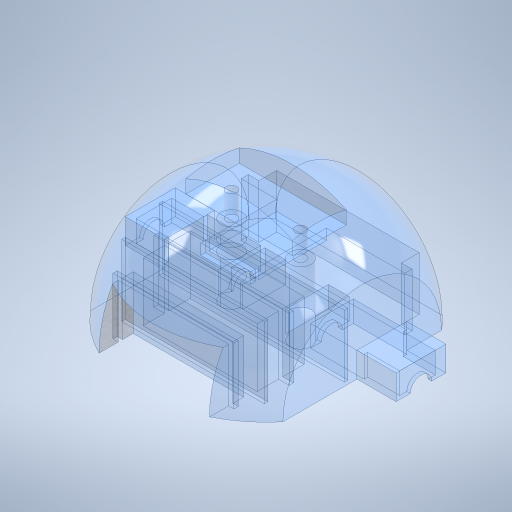
# Autodesk Inventor part: naibu-rightside
Saved by Autodesk Inventor 2023 (Build 270158000, 158)
## iProperties
Created: 2022-10-08
Part Number: naibu-rightside
Material: ABS プラスチック
Document SubType Name: Modeling
Designer: ellie
Density: 1.06 g/cm^3
Appearance: 青 - 光沢
Author: ellie
Autodesk Inventor part; units mm, degrees
ref_plane "YZ Plane" through (0, 0, 0) normal (1, 0, 0) x (0, 1, 0)
sketch "スケッチ1" plane through (0, 0, 0) normal (0, 1, 0) x (-1, 0, 0)
  circle A0 centre (0, 0) radius 35
  line L0 (0, 0) -> (0, -35)
  line L1 (0, 0) -> (0, 35)
  dimension "d0" = 70
  constraints: 4 end point, 2 point on circle, 2 vertical, 1 centre point, 1 coincident
  measures "d0" diameter of A0
revolve "回転1" add sketch "スケッチ1" angle 180 about axis through (0, 0, 0) along (0, 0, 1) picked at (-2.5961, -23.0408) contours L1 L0 A0
sketch "スケッチ5" plane through (0, 0, 0) normal (0, -1, 0) x (1, 0, 0)
  line L0 (-20, -23) -> (20, -23)
  line L1 (20, -23) -> (20, -16)
  line L2 (20, -16) -> (-20, -16)
  line L3 (-20, -16) -> (-20, -23)
  line L4 (-20, -16) -> (-23, -16)
  line L5 (-23, -16) -> (-23, -18)
  line L6 (-23, -18) -> (-20, -18)
  line L7 (-20, -18) -> (-20, -16)
  line L8 (0, 26) -> (-17, 26)
  line L9 (-17, 26) -> (-17, 24.8)
  line L10 (-17, 24.8) -> (0, 24.8)
  line L11 (0, 24.8) -> (0, 26)
  line L12 (0, 20.5) -> (-20, 20.5)
  line L13 (-20, 20.5) -> (-20, 19.5)
  line L14 (-20, 19.5) -> (0, 19.5)
  line L15 (0, 19.5) -> (0, 20.5)
  line L16 (0, 12.5) -> (-19, 12.5)
  line L17 (-19, 12.5) -> (-19, 11.3)
  line L18 (-19, 11.3) -> (0, 11.3)
  line L19 (0, 11.3) -> (0, 12.5)
  line L20 (0, 4) -> (-26, 4)
  line L21 (-26, 4) -> (-26, 3)
  line L22 (-26, 3) -> (0, 3)
  line L23 (0, 3) -> (0, 4)
  circle A0 centre (0, 0) radius 35 projected
  circle A1 centre (0, 0) radius 35 projected
  line L24 (0, 35) -> (0, -35)
  line L25 (35, 0) -> (-35, 0)
  line L26 (-37, -0.5262) -> (-28, -0.5262)
  line L27 (-28, -0.5262) -> (-28, -10.5262)
  line L28 (-28, -10.5262) -> (-37, -10.5262)
  line L29 (-37, -10.5262) -> (-37, -0.5262)
  line L30 (-28, -8.0262) -> (-28, -0.5262)
  line L31 (-27, 22.2711) -> (-27, -22.2711)
  line L32 (-15.5, 26) -> (0, 26)
  line L33 (0, 26) -> (0, 35)
  line L34 (0, 35) -> (-15.5, 35)
  line L35 (-15.5, 35) -> (-15.5, 26)
  line L36 (-15.5, 24.8) -> (0, 24.8)
  line L37 (0, 24.8) -> (0, 21.8)
  line L38 (0, 21.8) -> (-15.5, 21.8)
  line L39 (-15.5, 21.8) -> (-15.5, 24.8)
  line L40 (-16, 12.5) -> (0, 12.5)
  line L41 (0, 12.5) -> (0, 18.5)
  line L42 (0, 18.5) -> (-16, 18.5)
  line L43 (-16, 18.5) -> (-16, 12.5)
  line L44 (-16, 11.3) -> (0, 11.3)
  line L45 (0, 11.3) -> (0, 5.3)
  line L46 (0, 5.3) -> (-16, 5.3)
  line L47 (-16, 5.3) -> (-16, 11.3)
  line L48 (-28, -5.5262) -> (-44.6865, -5.5262)
  line L49 (-28, -5.5262) -> (-12.8337, -5.5262)
  line L50 (-13, 0.4738) -> (-28, 0.4738)
  line L51 (-28, 0.4738) -> (-28, -11.5262)
  line L52 (-28, -11.5262) -> (-13, -11.5262)
  line L53 (-13, -11.5262) -> (-13, 0.4738)
  line L54 (-13, 0.4738) -> (-28, -11.5262) construction
  line L55 (-28, 0.4738) -> (-13, -11.5262) construction
  line L56 (-28, 1.4738) -> (-38, 1.4738)
  line L57 (-38, 1.4738) -> (-38, -12.5262)
  line L58 (-38, -12.5262) -> (-28, -12.5262)
  line L59 (-28, -12.5262) -> (-28, 1.4738)
  line L60 (-28, 1.4738) -> (-38, -12.5262) construction
  line L61 (-38, 1.4738) -> (-28, -12.5262) construction
  line L62 (-13, 0.4738) -> (-6, 0.4738)
  line L63 (-6, 0.4738) -> (-6, -11.5262)
  line L64 (-6, -11.5262) -> (-13, -11.5262)
  line L65 (-13, -11.5262) -> (-13, 0.4738)
  line L66 (-13, 0.4738) -> (-6, -11.5262) construction
  line L67 (-6, 0.4738) -> (-13, -11.5262) construction
  line L68 (-28, -0.5262) -> (-27, -0.5262)
  line L69 (-28, -10.5262) -> (-27, -10.5262)
  line L70 (-28, 1.4738) -> (-27, 1.4738)
  line L71 (-28, -12.5262) -> (-27, -12.5262)
  line L72 (23.4307, -26) -> (-23.4307, -26)
  line L73 (-13, 0.4738) -> (-11.8, 0.4738)
  line L74 (-11.8, 0.4738) -> (-11.8, -11.5262)
  line L75 (-11.8, -11.5262) -> (-13, -11.5262)
  line L76 (-13, -11.5262) -> (-13, 0.4738)
  line L77 (-5, 5.3) -> (-2, 5.3)
  line L78 (-2, 5.3) -> (-2, -5)
  line L79 (-4, -7) -> (-5, -7)
  line L80 (-5, -2) -> (-5, 5.3)
  line L81 (-5, -7) -> (-6, -7)
  arc A2 (-6, -3.7321) -> (-5, -2) centre (-7, -2) ccw
  arc A3 (-4, -7) -> (-2, -5) centre (-4, -5) ccw
  line L82 (-16.5791, -16) -> (-13, -16)
  point P0 (0, -23)
  point P1 (0, -16)
  point P2 (0, 25.4)
  point P3 (0, 20)
  point P4 (0, 11.9)
  point P5 (0, 3.5)
  point P6 (-20, -19.5)
  point P7 (-27, -0.5262)
  point P8 (-27, -10.5262)
  point P9 (-15.5, 23.3)
  point P10 (-15.5, 31.3807)
  point P11 (0, 26)
  point P12 (0, 24.8)
  point P13 (0, 11.3)
  point P14 (0, 12.5)
  point P15 (-27, 0)
  point P16 (-29, 0)
  point P17 (-20, 0)
  point P18 (-20.5, -5.5262)
  point P19 (-33, -5.5262)
  point P20 (-9.5, -5.5262)
  point P21 (-27, 0.4738)
  point P22 (-27, -11.5262)
  point P23 (-13, 0)
  point P24 (-6, 0)
  point P25 (-2, -7)
  point P26 (-4.5, -7)
  point P27 (-5, 4)
  point P28 (-2, 4)
  point P29 (-2, 5.3)
  point P30 (-2, 3)
  point P31 (-5, 3)
  dimension "d12" = 40
  dimension "d13" = 7
  dimension "d21" = 3
  dimension "d22" = 2
  dimension "d23" = 17
  dimension "d24" = 1.2
  dimension "d27" = 20
  dimension "d28" = 1
  dimension "d30" = 19
  dimension "d31" = 1.2
  dimension "d33" = 1
  dimension "d88" = 0
  dimension "d89" = 0
  dimension "d90" = 12
  dimension "d92" = 20
  dimension "d93" = 9
  dimension "d94" = 14.5
  dimension "d95" = 22.5
  dimension "d96" = 31
  dimension "d97" = 9
  dimension "d98" = 10
  dimension "d113" = 27
  dimension "d122" = 15.5
  dimension "d123" = 35
  dimension "d124" = 3
  dimension "d125" = 15.5
  dimension "d126" = 6
  dimension "d127" = 6
  dimension "d128" = 16
  dimension "d129" = 16
  dimension "d137" = 26
  dimension "d147" = 12
  dimension "d148" = 2.5262
  dimension "d149" = 13
  dimension "d151" = 15
  dimension "d161" = 14
  dimension "d162" = 10
  dimension "d164" = 12
  dimension "d165" = 7
  dimension "d170" = 26
  dimension "d175" = 1.2
  dimension "d178" = 1
  dimension "d180" = 10
  dimension "d185" = 3
  dimension "d186" = 2
  dimension "d187" = 1
  dimension "d188" = 5
  constraints: 164 end point, 33 parallel, 20 horizontal, 19 perpendicular, 19 point on line, 16 midpoint, 5 collinear, 4 point on circle, 3 tangent, 2 centre point, 1 equal radius, 1 vertical, 20 other
  measures "d12" distance of L2.end L1.end
  measures "d13" distance of L1.end L0.end
  measures "d21" distance of L6.end L5.end
  measures "d22" distance of L5.end L4.end
  measures "d23" distance of L10.end L9.end
  measures "d24" distance of L9.end L8.end
  measures "d27" distance of L14.end L13.end
  measures "d28" distance of L13.end L12.end
  measures "d30" distance of L18.end L17.end
  measures "d31" distance of L17.end L16.end
  measures "d33" distance of L21.end L20.end
  measures "d89" distance from line of point (0, 0) L25
  measures "d90" distance from line of L0 point (0, -35)
  measures "d92" distance of the line from the sketch origin of L3
  measures "d93" distance from line of L8 point (0, 35)
  measures "d94" distance from line of L12 point (0, 35)
  measures "d95" distance from line of L16 point (0, 35)
  measures "d96" distance from line of L20 point (0, 35)
  measures "d97" distance of L27.end L28.end
  measures "d98" distance of L26.end L27.end
  measures "d113" distance of the line from the sketch origin of L31
  measures "d122" distance of the line from the sketch origin of L35
  measures "d123" distance between parallel lines of L34 L25
  measures "d124" distance of L36.end L37.end
  measures "d126" distance of L41.end L40.end
  measures "d127" distance of L44.end L45.end
  measures "d128" distance of the line from the sketch origin of L47
  measures "d129" distance of the line from the sketch origin of L43
  measures "d137" distance of L21.end L22.end
  measures "d147" distance of L51.end L50.end
  measures "d148" distance between parallel lines of L50 L22
  measures "d149" distance of the line from the sketch origin of L53
  measures "d151" distance between parallel lines of L53 L27
  measures "d161" distance between parallel lines of L58 L56
  measures "d162" distance between parallel lines of L51 L57
  measures "d164" distance between parallel lines of L64 L62
  measures "d165" distance between parallel lines of L53 L63
  measures "d170" distance between parallel lines of L72 L25
  measures "d175" distance of L74.end L75.end
  measures "d178" distance of L81.start L81.end
  measures "d180" distance between parallel lines of L81 L22
  measures "d185" distance of point (-2, -7) L79.end
  measures "d186" radius of A2
  measures "d187" distance between parallel lines of L80 L63
  measures "d188" distance from line of L81 A2.centre
extrude "GNSボード" cut sketch "スケッチ5" against normal blind 16 contours L11 L10 L9 L8
extrude "GNSボード止めるよう" cut sketch "スケッチ5" against normal blind 15 contours L24 L8 L35 A0 | L24 L38 L39 L10
extrude "アルミ板１" cut sketch "スケッチ5" against normal blind 20 contours L15 L14 L13 L12
extrude "メイン基板" cut sketch "スケッチ5" against normal blind 17.5 contours L18 L17 L16 L19
extrude "メイン止めるよう" cut sketch "スケッチ5" against normal blind 16.5 contours L46 L47 L18 L24 | L16 L43 L42 L24
extrude "アルミ板２" cut sketch "スケッチ5" against normal blind 17.5 contours L22 L78 L20 L23 | L22 L80 L20 L78 | L22 L21 L20 L80
extrude "電池ボックス入れ" cut sketch "スケッチ5" against normal blind 15 contours L3 L2 L24 L0 | L24 L2 L1 L0 | L6 L5 L4 L3
extrude "side ut" cut sketch "スケッチ5" against normal blind 100 contours A0 L58 L71 L31 | A0 L28 L51 L59 L58 | L71 L59 L52 L31 | A0 L48 L27 L28 | L52 L51 L69 L31 | L31 L70 L56 A0 | A0 L26 L27 L48 | L27 L49 L31 L69 | L56 L59 L51 L25 A0 | L31 L50 L59 L70 | A0 L25 L51 L26 | L27 L68 L31 L49 | L31 L25 L51 L50 | L31 L68 L51 L25
extrude "motor case" add sketch "スケッチ5" against normal blind 7 contours L58 L57 L48 L29 L28 A0 | A0 L28 L51 L59 L58 | L71 L59 L52 L31 | L28 L29 L48 A0 | A0 L48 L27 L28 | L52 L51 L69 L31 | L31 L49 L53 L52 | L48 L29 L26 A0 | A0 L26 L27 L48 | L27 L49 L31 L69 | L57 L56 A0 L26 L29 L48 | L56 L59 L51 L25 A0 | L31 L50 L59 L70 | L53 L49 L31 L25 | L25 L31 L50 L53 | A0 L25 L51 L26 | L27 L68 L31 L49 | L31 L25 L51 L50 | L31 L68 L51 L25
extrude "bottom cut" cut sketch "スケッチ5" against normal blind 90 contours L72 A0 L24 | L24 A0 L72
extrude "motor" cut sketch "スケッチ5" against normal blind 6 contours L63 L64 L74 L25 | L25 L74 L62 L63 | L28 L29 L48 A0 | A0 L48 L27 L28 | L52 L51 L69 L31 | L31 L49 L53 L52 | L74 L64 L53 L25 | L25 L53 L62 L74 | L48 L29 L26 A0 | A0 L26 L27 L48 | L27 L49 L31 L69 | L53 L49 L31 L25 | L25 L31 L50 L53 | L27 L68 L31 L49 | L31 L25 L51 L50 | L31 L68 L51 L25
extrude "motor block" add sketch "スケッチ5" against normal blind 10 contours L74 L64 L53 L25 | L25 L53 L62 L74
sketch "スケッチ26" plane through (-38, 0, -12.5262) normal (-1, 0, 0) x (0, 0, 1)
  line L0 (14, 0) -> (0, 0) projected
  circle A0 centre (7, 0) radius 3
  point P0 (12.5262, 0)
  point P1 (7, 0)
  point P2 (4, 0)
  point P3 (10, 0)
  dimension "d197" = 6
  constraints: 1 centre point, 1 coincident
  measures "d197" diameter of A0
extrude "押し出し34" cut sketch "スケッチ26" against normal blind 27 contours L0 A0 picked at (7.7485, 0.6631)
mirror "ミラー11" about plane through (0, 0, 0) normal (1, 0, 0) of "GNSボード", "GNSボード止めるよう", "アルミ板１", "メイン止めるよう", "メイン基板", "アルミ板２", "motor", "押し出し34", "motor case", "電池ボックス入れ", "motor block", "side ut"
ref_plane "作業平面5" through (0, 15, 0) normal (0, -1, 0) x (1, 0, 0)
sketch "スケッチ28" plane through (0, 15, 0) normal (0, -1, 0) x (1, 0, 0)
  line L0 (23, -16) -> (-23, -16) projected
  line L1 (-23, -18) -> (-23, -16) projected
  line L2 (-20, -18) -> (-23, -18) projected
  line L3 (-20, -23) -> (-20, -18) projected
  line L4 (20, -23) -> (-20, -23) projected
  line L5 (20, -18) -> (20, -23) projected
  line L6 (20, -18) -> (23, -18) projected
  line L7 (23, -18) -> (23, -16) projected
  line L8 (-13, -11.5262) -> (-13, 0.4738) projected
  line L9 (-28, 0.4738) -> (-13, 0.4738) projected
  line L10 (-28, -0.5262) -> (-28, 0.4738) projected
  line L11 (-37, -0.5262) -> (-28, -0.5262) projected
  line L12 (-37, -10.5262) -> (-37, -0.5262) projected
  line L13 (-28, -10.5262) -> (-37, -10.5262) projected
  line L14 (-28, -11.5262) -> (-28, -10.5262) projected
  line L15 (-13, -11.5262) -> (-28, -11.5262) projected
  line L16 (-11.8, 0.4738) -> (-11.8, -11.5262) projected
  line L17 (-6, -11.5262) -> (-11.8, -11.5262) projected
  line L18 (-6, 0.4738) -> (-6, -11.5262) projected
  line L19 (-11.8, 0.4738) -> (-6, 0.4738) projected
  arc A0 (-6, -3.7321) -> (-5, -2) centre (-7, -2) ccw projected
  line L20 (-5, -2) -> (-5, 5.3) projected
  line L21 (-2, 5.3) -> (-2, -5) projected
  arc A1 (-4, -7) -> (-2, -5) centre (-4, -5) ccw projected
  line L22 (-5, -7) -> (-6, -7) projected
  line L23 (-4, -7) -> (-5, -7) projected
  line L24 (-13, 5.3) -> (1, 5.3)
  line L25 (1, 5.3) -> (1, -16)
  line L26 (1, -16) -> (-13, -16)
  line L27 (-13, -16) -> (-13, 5.3)
  line L28 (-16, 5.3) -> (-16, 11.3) projected
  line L29 (0, 5.3) -> (-16, 5.3) projected
  line L30 (16, 5.3) -> (-16, 5.3) projected
  point P0 (0, 0)
  dimension "d198" = 14
  dimension "d199" = 3
  constraints: 8 end point, 2 parallel, 1 collinear, 1 horizontal, 1 perpendicular, 1 point on line
  measures "d198" distance of L25.end L26.end
  measures "d199" distance between parallel lines of L27 L28
extrude "押し出し35" cut sketch "スケッチ28" along normal blind 3 contours L0 L27 L8 L24 L20 A0 L18 L19 L16 L17 L22 L23 A1 L21 L25 | L21 A1 L23 L22 L18 A0 L20 L24 | L18 L17 L16 L19
ref_plane "作業平面6" through (-15.5, 35, 26) normal (0, -1, 0) x (1, 0, 0)
sketch "スケッチ29" plane through (-15.5, 35, 26) normal (0, -1, 0) x (1, 0, 0)
  line L0 (15.5, -26) -> (-67.7134, -26)
  line L1 (-67.7134, -26) -> (15.5, -26)
  line L2 (110.7852, -24.5555) -> (110.7852, -27.3413)
  line L3 (15.5, -26) -> (98.1975, -26)
  circle A0 centre (25.2, -26) radius 1.5
  circle A1 centre (5.8, -26) radius 1.5
  line L4 (32.5, 0) -> (-1.5, 0) projected
  line L5 (15.5, 0) -> (15.5, -52)
  line L6 (-7.9307, -52) -> (38.9307, -52) projected
  dimension "d205" = 3
  dimension "d206" = 19.4
  dimension "d207" = 0
  constraints: 10 end point, 2 centre point, 2 horizontal, 2 midpoint, 1 collinear, 1 vertical, 1 other
  measures "d205" diameter of A0
  measures "d206" distance of A1.centre A0.centre
  measures "d207" distance from line of L3 A0.centre
extrude "押し出し36" cut sketch "スケッチ29" along normal up to surface (35 mm away)
sketch "スケッチ30" plane through (-15.5, 35, 26) normal (0, -1, 0) x (1, 0, 0)
  line L0 (0.5, -18.5) -> (30.5, -18.5)
  line L1 (30.5, -18.5) -> (30.5, -33.5)
  line L2 (30.5, -33.5) -> (0.5, -33.5)
  line L3 (0.5, -33.5) -> (0.5, -18.5)
  line L4 (0.5, -18.5) -> (30.5, -33.5) construction
  line L5 (30.5, -18.5) -> (0.5, -33.5) construction
  point P0 (15.5, -26)
  dimension "d210" = 30
  dimension "d211" = 15
  constraints: 12 end point, 2 midpoint, 2 parallel, 1 horizontal, 1 perpendicular
  measures "d210" distance of L1.end L2.end
  measures "d211" distance of L0.end L1.end
extrude "押し出し37" cut sketch "スケッチ30" along normal blind 8
sketch "スケッチ31" plane through (-15.5, 0, 26) normal (0, -1, 0) x (1, 0, 0)
  arc A0 (4.3768, -25.5262) -> (7.2232, -25.5262) centre (5.8, -26) ccw projected
  circle A1 centre (5.8, -26) radius 3
  circle A2 centre (25.2, -26) radius 1.5 projected
  circle A3 centre (25.2, -26) radius 3
  point P0 (15.5, -26)
  dimension "d214" = 6
  dimension "d215" = 6
  constraints: 2 centre point, 2 coincident
  measures "d214" diameter of A1
  measures "d215" diameter of A3
extrude "押し出し38" cut sketch "スケッチ31" against normal blind 20 contours A1 | A2 | A3
